Autodesk Fusion 360 part; units mm, degrees
(part 3 of 4)
sketch "Sketch19" plane through (0, 0, 6.5) normal (0, 0, 1) x (-1, 0, 0)
  line L0 (61.5, -17) -> (61.5, 17)
  arc A0 (63.5, 19) -> (61.5, 17) centre (63.5, 17) ccw
  line L1 (63.5, 19) -> (68.5, 19)
  arc A1 (70.5, 17) -> (68.5, 19) centre (68.5, 17) ccw
  line L2 (70.5, 17) -> (70.5, -17)
  arc A2 (68.5, -19) -> (70.5, -17) centre (68.5, -17) ccw
  line L3 (68.5, -19) -> (63.5, -19)
  arc A3 (61.5, -17) -> (63.5, -19) centre (63.5, -17) ccw
  line L4 (59.5, 16.3) -> (20.05, 16.3)
  line L5 (20.05, 16.3) -> (20.05, 38.6)
  arc A4 (20.05, 38.6) -> (18.05, 40.6) centre (18.05, 38.6) ccw
  line L6 (18.05, 40.6) -> (-18.05, 40.6)
  arc A5 (-18.05, 40.6) -> (-20.05, 38.6) centre (-18.05, 38.6) ccw
  line L7 (-20.05, 38.6) -> (-20.05, 16.3)
  line L8 (-20.05, 16.3) -> (-72.5, 16.3)
  line L9 (-72.5, 16.3) -> (-72.5, -16.3)
  line L10 (-72.5, -16.3) -> (-20.05, -16.3)
  line L11 (-20.05, -16.3) -> (-20.05, -38.6)
  arc A6 (-20.05, -38.6) -> (-18.05, -40.6) centre (-18.05, -38.6) ccw
  line L12 (-18.05, -40.6) -> (18.05, -40.6)
  arc A7 (18.05, -40.6) -> (20.05, -38.6) centre (18.05, -38.6) ccw
  line L13 (20.05, -38.6) -> (20.05, -16.3)
  line L14 (20.05, -16.3) -> (59.5, -16.3)
  line L15 (59.5, -16.3) -> (59.5, -28.9174)
  arc A8 (61.5, -28.5) -> (59.5, -28.9174) centre (61.5, -33.5) ccw
  line L16 (61.5, -28.5) -> (72.5, -28.5)
  line L17 (72.5, -28.5) -> (72.5, 28.5)
  line L18 (72.5, 28.5) -> (61.5, 28.5)
  arc A9 (59.5, 28.9174) -> (61.5, 28.5) centre (61.5, 33.5) ccw
  line L19 (59.5, 28.9174) -> (59.5, 16.3)
  circle A10 centre (-10, 34.75) radius 2.425
  circle A11 centre (10, -34.75) radius 2.425
  circle A12 centre (-10, -34.75) radius 2.425
  circle A13 centre (10, 34.75) radius 2.425
  line L20 (59.5, -8.8707) -> (59.5, 8.8707)
  line L21 (-70.5, -8.9444) -> (-70.5, 8.9444)
  line L22 (55.628, -14.3) -> (-65.7592, -14.3)
  line L23 (55.628, 14.3) -> (-65.7592, 14.3)
  line L24 (55.7295, 13.3104) -> (1.8744, 2.1388)
  line L25 (-1.8855, 2.081) -> (-65.8457, 13.3075)
  line L26 (-68.1756, 10.918) -> (-4.7518, 0.4934)
  line L27 (-4.7518, -0.4934) -> (-68.1756, -10.918)
  line L28 (-65.8457, -13.3075) -> (-1.8855, -2.081)
  line L29 (1.8744, -2.1388) -> (55.7295, -13.3104)
  line L30 (57.1159, -10.8335) -> (4.2578, -0.4907)
  line L31 (4.2578, 0.4907) -> (57.1159, 10.8335)
  arc A14 (55.628, -14.3) -> (55.7295, -13.3104) centre (55.628, -13.8) ccw
  arc A15 (-65.8457, -13.3075) -> (-65.7592, -14.3) centre (-65.7592, -13.8) ccw
  arc A16 (-65.7592, 14.3) -> (-65.8457, 13.3075) centre (-65.7592, 13.8) ccw
  arc A17 (55.7295, 13.3104) -> (55.628, 14.3) centre (55.628, 13.8) ccw
  arc A18 (57.1159, -10.8335) -> (59.5, -8.8707) centre (57.5, -8.8707) ccw
  arc A19 (59.5, 8.8707) -> (57.1159, 10.8335) centre (57.5, 8.8707) ccw
  arc A20 (-68.1756, 10.918) -> (-70.5, 8.9444) centre (-68.5, 8.9444) ccw
  arc A21 (-70.5, -8.9444) -> (-68.1756, -10.918) centre (-68.5, -8.9444) ccw
  arc A22 (-1.8855, 2.081) -> (1.8744, 2.1388) centre (-0.1567, 11.9304) ccw
  arc A23 (1.8744, -2.1388) -> (-1.8855, -2.081) centre (-0.1567, -11.9304) ccw
  arc A24 (-4.7518, -0.4934) -> (-4.7518, 0.4934) centre (-4.8329, 0) ccw
  arc A25 (4.2578, 0.4907) -> (4.2578, -0.4907) centre (4.3538, 0) ccw
  point P0 (-70.5, -11.3)
  point P1 (-70.5, 11.3)
  point P2 (60.5, 14.3)
  point P3 (-71.5, 14.3)
  point P4 (0, 1.75)
  point P5 (-1.75, 0)
  point P6 (0, -1.75)
  point P7 (1.75, 0)
  dimension "d143" = 2
  dimension "d144" = 2
  dimension "d145" = 5
  dimension "d146" = 5
  dimension "d147" = 2
  dimension "d148" = 2
  dimension "d149" = 1
  dimension "d150" = 1
  dimension "d151" = 3.5
  dimension "d152" = 3.5
  dimension "d153" = 1.75
  dimension "d154" = 1.75
  dimension "d155" = 0.5
  dimension "d156" = 2
  dimension "d157" = 10
  dimension "d158" = 0.5
  constraint perpendicular L14 L20
  constraint perpendicular L8 L21
  constraint perpendicular L15 L22
  constraint perpendicular L21 L23
  constraint vertical P4 P6
  constraint vertical origin P4
  constraint horizontal P5 P7
  constraint horizontal origin P7
  constraint tangent L22 A14
  constraint tangent L29 A14
  constraint tangent L28 A15
  constraint tangent L22 A15
  constraint equal A14 A15
  constraint coincident P3 L25
  constraint coincident P3 L23
  constraint tangent L25 A16
  constraint tangent L23 A16
  constraint equal A14 A16
  constraint coincident P2 L23
  constraint coincident P2 L24
  constraint tangent L23 A17
  constraint tangent L24 A17
  constraint equal A14 A17
  constraint tangent L30 A18
  constraint tangent L20 A18
  constraint tangent L20 A19
  constraint tangent L31 A19
  constraint equal A18 A19
  constraint coincident P1 L26
  constraint coincident P1 L21
  constraint tangent L26 A20
  constraint tangent L21 A20
  constraint equal A18 A20
  constraint coincident P0 L21
  constraint coincident P0 L27
  constraint tangent L21 A21
  constraint tangent L27 A21
  constraint equal A18 A21
  constraint tangent L24 A22
  constraint tangent L25 A22
  constraint tangent L29 A23
  constraint tangent L28 A23
  constraint equal A22 A23
  constraint tangent L27 A24
  constraint tangent L26 A24
  constraint tangent L31 A25
  constraint tangent L30 A25
  constraint equal A24 A25
  measures "d143" distance of L0 L20
  measures "d144" distance of L9 L21
  measures "d145" distance of L10 P0
  measures "d146" distance of L8 P1
  measures "d147" distance of L4 L23
  measures "d148" distance of L14 L22
  measures "d149" distance of L9 P3
  measures "d150" distance of L0 P2
  measures "d151" distance of P4 P6
  measures "d152" distance of P5 P7
  measures "d153" distance of origin P4
  measures "d154" distance of origin P5
  measures "d155" radius of A14
  measures "d157" radius of A22
  measures "d158" radius of A24
extrude "Extrude21" cut sketch "Sketch19" against normal blind 6.5 contours L20 L30 L31 A18 A19 A25 | L21 L26 L27 A20 A21 A24 | L22 L28 L29 A14 A15 A23 | L23 L24 L25 A16 A17 A22
sketch "Sketch20" plane through (0, 0, 6.5) normal (0, 0, 1) x (-1, 0, 0)
  line L0 (-4.7518, -0.4934) -> (-68.1756, -10.918)
  arc A0 (-70.5, -8.9444) -> (-68.1756, -10.918) centre (-68.5, -8.9444) ccw
  line L1 (-70.5, -8.9444) -> (-70.5, 8.9444)
  arc A1 (-68.1756, 10.918) -> (-70.5, 8.9444) centre (-68.5, 8.9444) ccw
  line L2 (-68.1756, 10.918) -> (-4.7518, 0.4934)
  arc A2 (-4.7518, -0.4934) -> (-4.7518, 0.4934) centre (-4.8329, 0) ccw
  line L3 (59.5, 8.8707) -> (59.5, -8.8707)
  arc A3 (57.1159, -10.8335) -> (59.5, -8.8707) centre (57.5, -8.8707) ccw
  line L4 (57.1159, -10.8335) -> (4.2578, -0.4907)
  arc A4 (4.2578, 0.4907) -> (4.2578, -0.4907) centre (4.3538, 0) ccw
  line L5 (4.2578, 0.4907) -> (57.1159, 10.8335)
  arc A5 (59.5, 8.8707) -> (57.1159, 10.8335) centre (57.5, 8.8707) ccw
  line L6 (-65.7592, 14.3) -> (55.628, 14.3)
  arc A6 (55.7295, 13.3104) -> (55.628, 14.3) centre (55.628, 13.8) ccw
  line L7 (55.7295, 13.3104) -> (1.8744, 2.1388)
  arc A7 (-1.8855, 2.081) -> (1.8744, 2.1388) centre (-0.1567, 11.9304) ccw
  line L8 (-1.8855, 2.081) -> (-65.8457, 13.3075)
  arc A8 (-65.7592, 14.3) -> (-65.8457, 13.3075) centre (-65.7592, 13.8) ccw
  line L9 (1.8744, -2.1388) -> (55.7295, -13.3104)
  arc A9 (55.628, -14.3) -> (55.7295, -13.3104) centre (55.628, -13.8) ccw
  line L10 (55.628, -14.3) -> (-65.7592, -14.3)
  arc A10 (-65.8457, -13.3075) -> (-65.7592, -14.3) centre (-65.7592, -13.8) ccw
  line L11 (-65.8457, -13.3075) -> (-1.8855, -2.081)
  arc A11 (1.8744, -2.1388) -> (-1.8855, -2.081) centre (-0.1567, -11.9304) ccw
  line L12 (61.5, -17) -> (61.5, 17)
  arc A12 (63.5, 19) -> (61.5, 17) centre (63.5, 17) ccw
  line L13 (63.5, 19) -> (68.5, 19)
  arc A13 (70.5, 17) -> (68.5, 19) centre (68.5, 17) ccw
  line L14 (70.5, 17) -> (70.5, -17)
  arc A14 (68.5, -19) -> (70.5, -17) centre (68.5, -17) ccw
  line L15 (68.5, -19) -> (63.5, -19)
  arc A15 (61.5, -17) -> (63.5, -19) centre (63.5, -17) ccw
  line L16 (59.5, 16.3) -> (20.05, 16.3)
  line L17 (20.05, 16.3) -> (20.05, 38.6)
  arc A16 (20.05, 38.6) -> (18.05, 40.6) centre (18.05, 38.6) ccw
  line L18 (18.05, 40.6) -> (-18.05, 40.6)
  arc A17 (-18.05, 40.6) -> (-20.05, 38.6) centre (-18.05, 38.6) ccw
  line L19 (-20.05, 38.6) -> (-20.05, 16.3)
  line L20 (-20.05, 16.3) -> (-72.5, 16.3)
  line L21 (-72.5, 16.3) -> (-72.5, -16.3)
  line L22 (-72.5, -16.3) -> (-20.05, -16.3)
  line L23 (-20.05, -16.3) -> (-20.05, -38.6)
  arc A18 (-20.05, -38.6) -> (-18.05, -40.6) centre (-18.05, -38.6) ccw
  line L24 (-18.05, -40.6) -> (18.05, -40.6)
  arc A19 (18.05, -40.6) -> (20.05, -38.6) centre (18.05, -38.6) ccw
  line L25 (20.05, -38.6) -> (20.05, -16.3)
  line L26 (20.05, -16.3) -> (59.5, -16.3)
  line L27 (59.5, -16.3) -> (59.5, -28.9174)
  arc A20 (61.5, -28.5) -> (59.5, -28.9174) centre (61.5, -33.5) ccw
  line L28 (61.5, -28.5) -> (72.5, -28.5)
  line L29 (72.5, -28.5) -> (72.5, 28.5)
  line L30 (72.5, 28.5) -> (61.5, 28.5)
  arc A21 (59.5, 28.9174) -> (61.5, 28.5) centre (61.5, 33.5) ccw
  line L31 (59.5, 28.9174) -> (59.5, 16.3)
  circle A22 centre (-10, 34.75) radius 2.425
  circle A23 centre (10, -34.75) radius 2.425
  circle A24 centre (-10, -34.75) radius 2.425
  circle A25 centre (10, 34.75) radius 2.425
  line L32 (16.05, 16.3) -> (-16.05, 16.3)
  line L33 (-18.05, 18.3) -> (-18.05, 28.325)
  line L34 (-16.05, 30.325) -> (-7.575, 30.325)
  line L35 (18.05, 28.325) -> (18.05, 18.3)
  line L36 (-7.575, -30.325) -> (-16.05, -30.325)
  line L37 (-18.05, -28.325) -> (-18.05, -18.3)
  line L38 (-16.05, -16.3) -> (16.05, -16.3)
  line L39 (18.05, -18.3) -> (18.05, -28.325)
  arc A26 (16.05, 16.3) -> (18.05, 18.3) centre (16.05, 18.3) ccw
  arc A27 (18.05, 28.325) -> (16.05, 30.325) centre (16.05, 28.325) ccw
  arc A28 (-16.05, 30.325) -> (-18.05, 28.325) centre (-16.05, 28.325) ccw
  arc A29 (-18.05, 18.3) -> (-16.05, 16.3) centre (-16.05, 18.3) ccw
  arc A30 (18.05, -18.3) -> (16.05, -16.3) centre (16.05, -18.3) ccw
  arc A31 (16.05, -30.325) -> (18.05, -28.325) centre (16.05, -28.325) ccw
  arc A32 (-18.05, -28.325) -> (-16.05, -30.325) centre (-16.05, -28.325) ccw
  arc A33 (-16.05, -16.3) -> (-18.05, -18.3) centre (-16.05, -18.3) ccw
  line L40 (5.575, -32.325) -> (5.575, -38.6)
  line L41 (3.575, -40.6) -> (-3.575, -40.6)
  line L42 (-5.575, -38.6) -> (-5.575, -32.325)
  arc A34 (-5.575, -32.325) -> (-7.575, -30.325) centre (-7.575, -32.325) ccw
  line L43 (16.05, -30.325) -> (7.575, -30.325)
  arc A35 (7.575, -30.325) -> (5.575, -32.325) centre (7.575, -32.325) ccw
  arc A36 (-5.575, -38.6) -> (-3.575, -40.6) centre (-3.575, -38.6) ccw
  arc A37 (3.575, -40.6) -> (5.575, -38.6) centre (3.575, -38.6) ccw
  line L44 (-5.575, 30.325) -> (5.575, 30.325)
  line L45 (5.575, 32.325) -> (5.575, 38.6)
  line L46 (3.575, 40.6) -> (-3.575, 40.6)
  line L47 (-5.575, 38.6) -> (-5.575, 32.325)
  arc A38 (-3.575, 40.6) -> (-5.575, 38.6) centre (-3.575, 38.6) ccw
  arc A39 (5.575, 38.6) -> (3.575, 40.6) centre (3.575, 38.6) ccw
  arc A40 (-7.575, 30.325) -> (-5.575, 32.325) centre (-7.575, 32.325) ccw
  line L48 (7.575, 30.325) -> (16.05, 30.325)
  arc A41 (5.575, 32.325) -> (7.575, 30.325) centre (7.575, 32.325) ccw
  line L49 (-67.5, 42.6) -> (51.5, 42.6)
  line L50 (51.5, -42.6) -> (-67.5, -42.6)
  dimension "d161" = 4.425
  dimension "d162" = 4.425
  dimension "d163" = 2
  dimension "d164" = 2
  dimension "d165" = 2
  dimension "d166" = 2
  dimension "d167" = 2
  dimension "d168" = 2
  dimension "d215" = 4.425
  dimension "d216" = 4.425
  dimension "d218" = 2
  dimension "d219" = 2
  dimension "d220" = 2
  dimension "d221" = 4.425
  dimension "d222" = 4.425
  dimension "d224" = 2
  dimension "d225" = 2
  dimension "d226" = 2
  dimension "d254" = 2
  dimension "d255" = 2
  constraint horizontal L32
  constraint vertical L33
  constraint horizontal L34
  constraint vertical L35
  constraint horizontal L36
  constraint vertical L37
  constraint horizontal L38
  constraint vertical L39
  constraint tangent L32 A26
  constraint tangent L35 A26
  constraint tangent L35 A27
  constraint tangent L34 A27
  constraint equal A26 A27
  constraint tangent L34 A28
  constraint tangent L33 A28
  constraint equal A26 A28
  constraint tangent L33 A29
  constraint tangent L32 A29
  constraint equal A26 A29
  constraint tangent L38 A30
  constraint tangent L39 A30
  constraint tangent L39 A31
  constraint tangent L36 A31
  constraint equal A30 A31
  constraint tangent L36 A32
  constraint tangent L37 A32
  constraint equal A30 A32
  constraint tangent L37 A33
  constraint tangent L38 A33
  constraint equal A30 A33
  constraint vertical L40
  constraint horizontal L41
  constraint vertical L42
  constraint coincident L36 A31.start
  constraint tangent L42 A34
  constraint tangent L36 A34
  constraint tangent A31 L43
  constraint tangent L40 A35
  constraint tangent L43 A35
  constraint tangent L42 A36
  constraint tangent L41 A36
  constraint tangent L41 A37
  constraint tangent L40 A37
  constraint equal A36 A37
  constraint horizontal L44
  constraint vertical L45
  constraint horizontal L46
  constraint vertical L47
  constraint coincident L34 L44.start
  constraint tangent L47 A38
  constraint tangent L46 A38
  constraint tangent L46 A39
  constraint tangent L45 A39
  constraint equal A38 A39
  constraint coincident L44.start L47
  constraint tangent L47 A40
  constraint tangent L34 A40
  constraint tangent A27 L48
  constraint coincident L44.end L45
  constraint coincident L44.end L48
  constraint tangent L45 A41
  constraint tangent L48 A41
  measures "d161" distance of A25.centre L34
  measures "d162" distance of A23.centre L36
  measures "d163" distance of L25 L39
  measures "d164" distance of L23 L37
  measures "d165" distance of L6 L32
  measures "d166" distance of L10 L38
  measures "d167" radius of A26
  measures "d168" radius of A30
  measures "d215" distance of A23.centre L40
  measures "d216" distance of A24.centre L42
  measures "d218" radius of A34
  measures "d219" radius of A35
  measures "d220" radius of A36
  measures "d221" distance of A25.centre L45
  measures "d222" distance of A22.centre L47
  measures "d224" radius of A38
  measures "d225" radius of A40
  measures "d226" radius of A41
  measures "d254" distance of L46 L49
  measures "d255" distance of L41 L50
extrude "Extrude22" cut sketch "Sketch20" against normal blind 6.5 contours L18 L32 L33 L34 L35 A26 A27 A28 A29 L45 L46 L47 A38 A39 A40 L48 A41 | L24 L36 L37 L38 L39 A30 A31 A32 A33 L40 L41 L42 A34 L43 A35 A36 A37
ref_plane "WorkPlane3" through (8, -36.725, 15) normal (0, 0, 1) x (1, 0, 0)
sketch "Sketch21" plane through (0, 0, 15) normal (0, 0, 1) x (1, 0, 0)
  line L0 (-41.4565, -30.974) -> (-24.05, -30.974)
  line L1 (-22.05, -32.974) -> (-22.05, -38.6)
  line L2 (-24.05, -40.6) -> (-41.4565, -40.6)
  line L3 (-43.4565, -38.6) -> (-43.4565, -32.974)
  line L4 (24.05, -30.974) -> (57.4565, -30.974)
  line L5 (59.4565, -32.974) -> (59.4565, -38.6)
  line L6 (57.4565, -40.6) -> (24.05, -40.6)
  line L7 (22.05, -38.6) -> (22.05, -32.974)
  line L8 (-41.4565, 40.6) -> (-24.05, 40.6)
  line L9 (-22.05, 38.6) -> (-22.05, 32.974)
  line L10 (-24.05, 30.974) -> (-41.4565, 30.974)
  line L11 (-43.4565, 32.974) -> (-43.4565, 38.6)
  line L12 (24.05, 40.6) -> (57.4565, 40.6)
  line L13 (59.4565, 38.6) -> (59.4565, 32.974)
  line L14 (57.4565, 30.974) -> (24.05, 30.974)
  line L15 (22.05, 32.974) -> (22.05, 38.6)
  line L16 (67.5, -42.6) -> (-51.5, -42.6)
  line L17 (-51.5, 42.6) -> (67.5, 42.6)
  line L18 (-20.05, -33.5) -> (-20.05, -38.6)
  line L19 (20.05, 33.5) -> (20.05, 38.6)
  line L20 (-56.5, -28.974) -> (-20.05, -28.974)
  line L21 (-20.05, 28.974) -> (-56.5, 28.974)
  circle A0 centre (-49, -35.1) radius 3.5435
  circle A1 centre (65, 35.1) radius 3.5435
  arc A2 (-41.4565, 40.6) -> (-43.4565, 38.6) centre (-41.4565, 38.6) ccw
  arc A3 (-22.05, 38.6) -> (-24.05, 40.6) centre (-24.05, 38.6) ccw
  arc A4 (-24.05, 30.974) -> (-22.05, 32.974) centre (-24.05, 32.974) ccw
  arc A5 (-43.4565, 32.974) -> (-41.4565, 30.974) centre (-41.4565, 32.974) ccw
  arc A6 (24.05, 40.6) -> (22.05, 38.6) centre (24.05, 38.6) ccw
  arc A7 (59.4565, 38.6) -> (57.4565, 40.6) centre (57.4565, 38.6) ccw
  arc A8 (57.4565, 30.974) -> (59.4565, 32.974) centre (57.4565, 32.974) ccw
  arc A9 (22.05, 32.974) -> (24.05, 30.974) centre (24.05, 32.974) ccw
  arc A10 (-41.4565, -30.974) -> (-43.4565, -32.974) centre (-41.4565, -32.974) ccw
  arc A11 (-22.05, -32.974) -> (-24.05, -30.974) centre (-24.05, -32.974) ccw
  arc A12 (-24.05, -40.6) -> (-22.05, -38.6) centre (-24.05, -38.6) ccw
  arc A13 (-43.4565, -38.6) -> (-41.4565, -40.6) centre (-41.4565, -38.6) ccw
  arc A14 (24.05, -30.974) -> (22.05, -32.974) centre (24.05, -32.974) ccw
  arc A15 (59.4565, -32.974) -> (57.4565, -30.974) centre (57.4565, -32.974) ccw
  arc A16 (57.4565, -40.6) -> (59.4565, -38.6) centre (57.4565, -38.6) ccw
  arc A17 (22.05, -38.6) -> (24.05, -40.6) centre (24.05, -38.6) ccw
  dimension "d172" = 2
  dimension "d173" = 2
  dimension "d174" = 2
  dimension "d175" = 2
  dimension "d176" = 2
  dimension "d177" = 2
  dimension "d178" = 5.5435
  dimension "d179" = 5.5435
  dimension "d180" = 2
  dimension "d181" = 2
  dimension "d182" = 2
  dimension "d183" = 2
  constraint horizontal L0
  constraint vertical L1
  constraint horizontal L2
  constraint vertical L3
  constraint horizontal L4
  constraint vertical L5
  constraint horizontal L6
  constraint vertical L7
  constraint horizontal L8
  constraint vertical L9
  constraint horizontal L10
  constraint vertical L11
  constraint horizontal L12
  constraint vertical L13
  constraint horizontal L14
  constraint vertical L15
  constraint tangent L8 A2
  constraint tangent L11 A2
  constraint tangent L8 A3
  constraint tangent L9 A3
  constraint equal A2 A3
  constraint tangent L9 A4
  constraint tangent L10 A4
  constraint equal A2 A4
  constraint tangent L10 A5
  constraint tangent L11 A5
  constraint equal A2 A5
  constraint tangent L15 A6
  constraint tangent L12 A6
  constraint tangent L12 A7
  constraint tangent L13 A7
  constraint equal A6 A7
  constraint tangent L13 A8
  constraint tangent L14 A8
  constraint equal A6 A8
  constraint tangent L14 A9
  constraint tangent L15 A9
  constraint equal A6 A9
  constraint tangent L3 A10
  constraint tangent L0 A10
  constraint tangent L0 A11
  constraint tangent L1 A11
  constraint equal A10 A11
  constraint tangent L1 A12
  constraint tangent L2 A12
  constraint equal A10 A12
  constraint tangent L2 A13
  constraint tangent L3 A13
  constraint equal A10 A13
  constraint tangent L7 A14
  constraint tangent L4 A14
  constraint tangent L4 A15
  constraint tangent L5 A15
  constraint equal A14 A15
  constraint tangent L5 A16
  constraint tangent L6 A16
  constraint equal A14 A16
  constraint tangent L6 A17
  constraint tangent L7 A17
  constraint equal A14 A17
  constraint vertical A8.centre A15.centre
  constraint vertical A9.centre A14.centre
  constraint horizontal A11.centre A14.centre
  constraint horizontal A12.centre A17.centre
  constraint vertical A4.centre A11.centre
  constraint vertical A5.centre A10.centre
  constraint horizontal A4.centre A9.centre
  constraint horizontal A3.centre A6.centre
  measures "d172" distance of L2 L16
  measures "d173" distance of L8 L17
  measures "d174" distance of L1 L18
  measures "d175" distance of L15 L19
  measures "d176" distance of L0 L20
  measures "d177" distance of L10 L21
  measures "d178" distance of L3 A0.centre
  measures "d179" distance of L13 A1.centre
  measures "d180" radius of A2
  measures "d181" radius of A6
  measures "d182" radius of A10
  measures "d183" radius of A14
extrude "Extrude23" cut sketch "Sketch21" against normal blind 15 contours L0 L1 L2 L3 A10 A11 A12 A13 | L4 L5 L6 L7 A14 A15 A16 A17 | L8 L9 L10 L11 A2 A3 A4 A5 | L12 L13 L14 L15 A6 A7 A8 A9
sketch "Sketch22" plane through (-72.5, 0, 0) normal (-1, 0, 0) x (0, -1, 0)
  line L0 (-28.5, 6.5) -> (-28.5, 0)
  line L1 (-28.5, 0) -> (28.5, 0)
  line L2 (28.5, 0) -> (28.5, 6.5)
  line L3 (28.5, 6.5) -> (-28.5, 6.5)
  line L4 (-18, 4.5) -> (18, 4.5)
  line L5 (19, 3.5) -> (19, 3)
  line L6 (18, 2) -> (-18, 2)
  line L7 (-19, 3) -> (-19, 3.5)
  arc A0 (-18, 4.5) -> (-19, 3.5) centre (-18, 3.5) ccw
  arc A1 (-19, 3) -> (-18, 2) centre (-18, 3) ccw
  arc A2 (18, 2) -> (19, 3) centre (18, 3) ccw
  arc A3 (19, 3.5) -> (18, 4.5) centre (18, 3.5) ccw
  dimension "d186" = 2
  dimension "d187" = 2
  dimension "d190" = 1
  dimension "d287" = 9.5
  dimension "d288" = 9.5
  constraint horizontal L4
  constraint vertical L5
  constraint horizontal L6
  constraint vertical L7
  constraint tangent L4 A0
  constraint tangent L7 A0
  constraint tangent L7 A1
  constraint tangent L6 A1
  constraint equal A0 A1
  constraint tangent L6 A2
  constraint tangent L5 A2
  constraint equal A0 A2
  constraint tangent L5 A3
  constraint tangent L4 A3
  constraint equal A0 A3
  measures "d186" distance of L3 L4
  measures "d187" distance of L1 L6
  measures "d190" radius of A0
  measures "d287" distance of L2 L5
  measures "d288" distance of L0 L7
extrude "Extrude24" cut sketch "Sketch22" against normal blind 5 contours L4 L5 L6 L7 A0 A1 A2 A3
sketch "Sketch23" plane through (-61.5, 0, 0) normal (-1, 0, 0) x (0, -1, 0)
  line L0 (17, 6.5) -> (-17, 6.5)
  line L1 (-17, 6.5) -> (-17, 0)
  line L2 (-17, 0) -> (17, 0)
  line L3 (17, 0) -> (17, 6.5)
  line L4 (-9, 4.5) -> (9, 4.5)
  line L5 (10, 3.5) -> (10, 3)
  line L6 (9, 2) -> (-9, 2)
  line L7 (-10, 3) -> (-10, 3.5)
  arc A0 (-9, 4.5) -> (-10, 3.5) centre (-9, 3.5) ccw
  arc A1 (-10, 3) -> (-9, 2) centre (-9, 3) ccw
  arc A2 (9, 2) -> (10, 3) centre (9, 3) ccw
  arc A3 (10, 3.5) -> (9, 4.5) centre (9, 3.5) ccw
  dimension "d193" = 20
  dimension "d194" = 10
  dimension "d195" = 2
  dimension "d196" = 2
  dimension "d197" = 1
  constraint horizontal L4
  constraint vertical L5
  constraint horizontal L6
  constraint vertical L7
  constraint tangent L4 A0
  constraint tangent L7 A0
  constraint tangent L7 A1
  constraint tangent L6 A1
  constraint equal A0 A1
  constraint tangent L6 A2
  constraint tangent L5 A2
  constraint equal A0 A2
  constraint tangent L5 A3
  constraint tangent L4 A3
  constraint equal A0 A3
  measures "d193" distance of L5 L7
  measures "d194" distance of origin L7
  measures "d195" distance of L2 L6
  measures "d196" distance of L0 L4
  measures "d197" radius of A0
extrude "Extrude25" cut sketch "Sketch23" against normal blind 5 contours L4 L5 L6 L7 A0 A1 A2 A3
sketch "Sketch24" plane through (72.5, 0, 0) normal (1, 0, 0) x (0, 1, 0)
  line L0 (37.6, 0) -> (37.6, 10)
  line L1 (37.6, 10) -> (33.5, 10)
  arc A0 (28.974, 12.875) -> (33.5, 10) centre (33.5, 15) ccw
  arc A1 (28.974, 12.875) -> (24.4481, 15.75) centre (24.4481, 10.75) ccw
  line L2 (24.4481, 15.75) -> (24.3, 15.75)
  arc A2 (24.3, 15.75) -> (19.3, 10.75) centre (24.3, 10.75) ccw
  line L3 (19.3, 10.75) -> (19.3, 9.5)
  arc A3 (16.3, 6.5) -> (19.3, 9.5) centre (16.3, 9.5) ccw
  line L4 (16.3, 6.5) -> (-16.3, 6.5)
  arc A4 (-19.3, 9.5) -> (-16.3, 6.5) centre (-16.3, 9.5) ccw
  line L5 (-19.3, 9.5) -> (-19.3, 10.75)
  arc A5 (-19.3, 10.75) -> (-24.3, 15.75) centre (-24.3, 10.75) ccw
  line L6 (-24.3, 15.75) -> (-24.4481, 15.75)
  arc A6 (-24.4481, 15.75) -> (-28.974, 12.875) centre (-24.4481, 10.75) ccw
  arc A7 (-33.5, 10) -> (-28.974, 12.875) centre (-33.5, 15) ccw
  line L7 (-33.5, 10) -> (-37.6, 10)
  line L8 (-37.6, 10) -> (-37.6, 0)
  line L9 (-37.6, 0) -> (37.6, 0)
  line L10 (-9, 4.5) -> (9, 4.5)
  line L11 (10, 3.5) -> (10, 3)
  line L12 (9, 2) -> (-9, 2)
  line L13 (-10, 3) -> (-10, 3.5)
  arc A8 (-9, 4.5) -> (-10, 3.5) centre (-9, 3.5) ccw
  arc A9 (-10, 3) -> (-9, 2) centre (-9, 3) ccw
  arc A10 (9, 2) -> (10, 3) centre (9, 3) ccw
  arc A11 (10, 3.5) -> (9, 4.5) centre (9, 3.5) ccw
  dimension "d200" = 2
  dimension "d201" = 2
  dimension "d202" = 10
  dimension "d203" = 20
  dimension "d204" = 1
  constraint horizontal L10
  constraint vertical L11
  constraint horizontal L12
  constraint vertical L13
  constraint tangent L10 A8
  constraint tangent L13 A8
  constraint tangent L13 A9
  constraint tangent L12 A9
  constraint equal A8 A9
  constraint tangent L12 A10
  constraint tangent L11 A10
  constraint equal A8 A10
  constraint tangent L11 A11
  constraint tangent L10 A11
  constraint equal A8 A11
  measures "d200" distance of L4 L10
  measures "d201" distance of L9 L12
  measures "d202" distance of origin L11
  measures "d203" distance of L11 L13
  measures "d204" radius of A8
extrude "Extrude26" cut sketch "Sketch24" against normal blind 5 contours L10 L11 L12 L13 A8 A9 A10 A11
sketch "Sketch25" plane through (0, 14.3, 0) normal (0, -1, 0) x (1, 0, 0)
  line L0 (65.7592, 6.5) -> (-55.628, 6.5)
  line L1 (-55.628, 6.5) -> (-55.628, 0)
  line L2 (-55.628, 0) -> (65.7592, 0)
  line L3 (65.7592, 0) -> (65.7592, 6.5)
  line L4 (-17.05, 4.5) -> (17.05, 4.5)
  line L5 (18.05, 3.5) -> (18.05, 3)
  line L6 (17.05, 2) -> (-17.05, 2)
  line L7 (-18.05, 3) -> (-18.05, 3.5)
  line L8 (67.5, 10) -> (-51.5, 10)
  arc A0 (-17.05, 4.5) -> (-18.05, 3.5) centre (-17.05, 3.5) ccw
  arc A1 (-18.05, 3) -> (-17.05, 2) centre (-17.05, 3) ccw
  arc A2 (17.05, 2) -> (18.05, 3) centre (17.05, 3) ccw
  arc A3 (18.05, 3.5) -> (17.05, 4.5) centre (17.05, 3.5) ccw
  dimension "d207" = 36.1
  dimension "d208" = 18.05
  dimension "d209" = 2
  dimension "d211" = 1
  dimension "d212" = 2
  constraint horizontal L4
  constraint vertical L5
  constraint horizontal L6
  constraint vertical L7
  constraint tangent L4 A0
  constraint tangent L7 A0
  constraint tangent L7 A1
  constraint tangent L6 A1
  constraint equal A0 A1
  constraint tangent L6 A2
  constraint tangent L5 A2
  constraint equal A0 A2
  constraint tangent L5 A3
  constraint tangent L4 A3
  constraint equal A0 A3
  measures "d207" distance of L5 L7
  measures "d208" distance of origin L5
  measures "d209" distance of L2 L6
  measures "d211" radius of A0
  measures "d212" distance of L0 L4
extrude "Extrude27" cut sketch "Sketch25" against normal blind 5 contours L4 L5 L6 L7 A0 A1 A2 A3
sketch "Sketch26" plane through (0, -14.3, 0) normal (0, 1, 0) x (-1, 0, 0)
  line L0 (55.628, 6.5) -> (-65.7592, 6.5)
  line L1 (-65.7592, 6.5) -> (-65.7592, 0)
  line L2 (-65.7592, 0) -> (55.628, 0)
  line L3 (55.628, 0) -> (55.628, 6.5)
  line L4 (-17.05, 4.5) -> (17.05, 4.5)
  line L5 (18.05, 3.5) -> (18.05, 3)
  line L6 (17.05, 2) -> (-17.05, 2)
  line L7 (-18.05, 3) -> (-18.05, 3.5)
  arc A0 (-17.05, 4.5) -> (-18.05, 3.5) centre (-17.05, 3.5) ccw
  arc A1 (18.05, 3.5) -> (17.05, 4.5) centre (17.05, 3.5) ccw
  arc A2 (17.05, 2) -> (18.05, 3) centre (17.05, 3) ccw
  arc A3 (-18.05, 3) -> (-17.05, 2) centre (-17.05, 3) ccw
  dimension "d227" = 2
  dimension "d228" = 2
  dimension "d229" = 36.1
  dimension "d230" = 18.05
  dimension "d231" = 1
  constraint horizontal L4
  constraint vertical L5
  constraint horizontal L6
  constraint vertical L7
  constraint tangent L7 A0
  constraint tangent L4 A0
  constraint tangent L4 A1
  constraint tangent L5 A1
  constraint equal A0 A1
  constraint tangent L5 A2
  constraint tangent L6 A2
  constraint equal A0 A2
  constraint tangent L6 A3
  constraint tangent L7 A3
  constraint equal A0 A3
  measures "d227" distance of L0 L4
  measures "d228" distance of L2 L6
  measures "d229" distance of L5 L7
  measures "d230" distance of origin L5
  measures "d231" radius of A0
extrude "Extrude28" cut sketch "Sketch26" against normal blind 5 contours L4 L5 L6 L7 A0 A1 A2 A3
sketch "Sketch27" plane through (0, -42.6, 0) normal (0, -1, 0) x (1, 0, 0)
  line L0 (67.5, 0) -> (67.5, 10)
  line L1 (67.5, 10) -> (-51.5, 10)
  line L2 (-51.5, 10) -> (-51.5, 0)
  line L3 (-51.5, 0) -> (67.5, 0)
  line L4 (-41.4565, 8) -> (-24.05, 8)
  line L5 (-22.05, 6) -> (-22.05, 4)
  line L6 (-24.05, 2) -> (-41.4565, 2)
  line L7 (-43.4565, 4) -> (-43.4565, 6)
  line L8 (24.05, 8) -> (57.4565, 8)
  line L9 (59.4565, 6) -> (59.4565, 4)
  line L10 (57.4565, 2) -> (24.05, 2)
  line L11 (22.05, 4) -> (22.05, 6)
  arc A0 (-41.4565, 8) -> (-43.4565, 6) centre (-41.4565, 6) ccw
  arc A1 (-43.4565, 4) -> (-41.4565, 2) centre (-41.4565, 4) ccw
  arc A2 (-24.05, 2) -> (-22.05, 4) centre (-24.05, 4) ccw
  arc A3 (-22.05, 6) -> (-24.05, 8) centre (-24.05, 6) ccw
  arc A4 (24.05, 8) -> (22.05, 6) centre (24.05, 6) ccw
  arc A5 (59.4565, 6) -> (57.4565, 8) centre (57.4565, 6) ccw
  arc A6 (57.4565, 2) -> (59.4565, 4) centre (57.4565, 4) ccw
  arc A7 (22.05, 4) -> (24.05, 2) centre (24.05, 4) ccw
  line L12 (-3.575, 8) -> (3.575, 8)
  line L13 (5.575, 6) -> (5.575, 4)
  line L14 (3.575, 2) -> (-3.575, 2)
  line L15 (-5.575, 4) -> (-5.575, 6)
  arc A8 (-3.575, 8) -> (-5.575, 6) centre (-3.575, 6) ccw
  arc A9 (5.575, 6) -> (3.575, 8) centre (3.575, 6) ccw
  arc A10 (3.575, 2) -> (5.575, 4) centre (3.575, 4) ccw
  arc A11 (-5.575, 4) -> (-3.575, 2) centre (-3.575, 4) ccw
  point P0 (-20.05, 10)
  point P1 (20.05, 10)
  dimension "d234" = 2
  dimension "d235" = 2
  dimension "d236" = 2
  dimension "d238" = 21.4065
  dimension "d241" = 2
  dimension "d242" = 2
  dimension "d243" = 2
  dimension "d244" = 2
  dimension "d245" = 37.4065
  dimension "d246" = 2
  dimension "d249" = 2
  dimension "d250" = 11.15
  dimension "d251" = 5.575
  constraint horizontal L4
  constraint vertical L5
  constraint horizontal L6
  constraint vertical L7
  constraint horizontal L8
  constraint vertical L9
  constraint horizontal L10
  constraint vertical L11
  constraint tangent L4 A0
  constraint tangent L7 A0
  constraint tangent L7 A1
  constraint tangent L6 A1
  constraint equal A0 A1
  constraint tangent L6 A2
  constraint tangent L5 A2
  constraint equal A0 A2
  constraint tangent L5 A3
  constraint tangent L4 A3
  constraint equal A0 A3
  constraint tangent L11 A4
  constraint tangent L8 A4
  constraint tangent L8 A5
  constraint tangent L9 A5
  constraint equal A4 A5
  constraint tangent L9 A6
  constraint tangent L10 A6
  constraint equal A4 A6
  constraint tangent L10 A7
  constraint tangent L11 A7
  constraint equal A4 A7
  constraint horizontal L12
  constraint vertical L13
  constraint horizontal L14
  constraint vertical L15
  constraint tangent L15 A8
  constraint tangent L12 A8
  constraint tangent L12 A9
  constraint tangent L13 A9
  constraint equal A8 A9
  constraint tangent L13 A10
  constraint tangent L14 A10
  constraint equal A8 A10
  constraint tangent L14 A11
  constraint tangent L15 A11
  constraint equal A8 A11
  constraint horizontal A2.centre A11.centre
  constraint horizontal A4.centre A9.centre
  measures "d234" distance of L5 P0
  measures "d235" distance of L1 L4
  measures "d236" distance of L3 L6
  measures "d238" distance of L5 L7
  measures "d241" radius of A0
  measures "d242" distance of L11 P1
  measures "d243" distance of L1 L8
  measures "d244" distance of L3 L10
  measures "d245" distance of L9 L11
  measures "d246" radius of A4
  measures "d249" radius of A8
  measures "d250" distance of L13 L15
  measures "d251" distance of origin L15
extrude "Extrude31" cut sketch "Sketch27" against normal blind 7 contours L4 L5 L6 L7 A0 A1 A2 A3 | L8 L9 L10 L11 A4 A5 A6 A7 | L12 L13 L14 L15 A8 A9 A10 A11
sketch "Sketch28" plane through (0, 42.6, 0) normal (0, 1, 0) x (-1, 0, 0)
  line L0 (51.5, 0) -> (51.5, 10)
  line L1 (51.5, 10) -> (-67.5, 10)
  line L2 (-67.5, 10) -> (-67.5, 0)
  line L3 (-67.5, 0) -> (51.5, 0)
  line L4 (-57.4565, 8) -> (-24.05, 8)
  line L5 (-22.05, 6) -> (-22.05, 4)
  line L6 (-24.05, 2) -> (-57.4565, 2)
  line L7 (-59.4565, 4) -> (-59.4565, 6)
  line L8 (-3.575, 8) -> (3.575, 8)
  line L9 (5.575, 6) -> (5.575, 4)
  line L10 (3.575, 2) -> (-3.575, 2)
  line L11 (-5.575, 4) -> (-5.575, 6)
  line L12 (24.05, 8) -> (41.4565, 8)
  line L13 (43.4565, 6) -> (43.4565, 4)
  line L14 (41.4565, 2) -> (24.05, 2)
  line L15 (22.05, 4) -> (22.05, 6)
  arc A0 (-57.4565, 8) -> (-59.4565, 6) centre (-57.4565, 6) ccw
  arc A1 (-22.05, 6) -> (-24.05, 8) centre (-24.05, 6) ccw
  arc A2 (-24.05, 2) -> (-22.05, 4) centre (-24.05, 4) ccw
  arc A3 (-59.4565, 4) -> (-57.4565, 2) centre (-57.4565, 4) ccw
  arc A4 (-3.575, 8) -> (-5.575, 6) centre (-3.575, 6) ccw
  arc A5 (5.575, 6) -> (3.575, 8) centre (3.575, 6) ccw
  arc A6 (3.575, 2) -> (5.575, 4) centre (3.575, 4) ccw
  arc A7 (-5.575, 4) -> (-3.575, 2) centre (-3.575, 4) ccw
  arc A8 (24.05, 8) -> (22.05, 6) centre (24.05, 6) ccw
  arc A9 (43.4565, 6) -> (41.4565, 8) centre (41.4565, 6) ccw
  arc A10 (41.4565, 2) -> (43.4565, 4) centre (41.4565, 4) ccw
  arc A11 (22.05, 4) -> (24.05, 2) centre (24.05, 4) ccw
  point P0 (-20.05, 10)
  point P1 (20.05, 10)
  dimension "d256" = 2
  dimension "d257" = 2
  dimension "d258" = 2
  dimension "d259" = 37.4065
  dimension "d260" = 2
  dimension "d261" = 2
  dimension "d262" = 2
  dimension "d263" = 21.4065
  dimension "d264" = 2
  dimension "d265" = 11.15
  dimension "d266" = 5.575
  constraint horizontal L4
  constraint vertical L5
  constraint horizontal L6
  constraint vertical L7
  constraint horizontal L8
  constraint vertical L9
  constraint horizontal L10
  constraint vertical L11
  constraint horizontal L12
  constraint vertical L13
  constraint horizontal L14
  constraint vertical L15
  constraint tangent L7 A0
  constraint tangent L4 A0
  constraint tangent L4 A1
  constraint tangent L5 A1
  constraint equal A0 A1
  constraint tangent L5 A2
  constraint tangent L6 A2
  constraint equal A0 A2
  constraint tangent L6 A3
  constraint tangent L7 A3
  constraint equal A0 A3
  constraint tangent L11 A4
  constraint tangent L8 A4
  constraint tangent L8 A5
  constraint tangent L9 A5
  constraint equal A4 A5
  constraint tangent L9 A6
  constraint tangent L10 A6
  constraint equal A4 A6
  constraint tangent L10 A7
  constraint tangent L11 A7
  constraint equal A4 A7
  constraint tangent L15 A8
  constraint tangent L12 A8
  constraint tangent L12 A9
  constraint tangent L13 A9
  constraint equal A8 A9
  constraint tangent L13 A10
  constraint tangent L14 A10
  constraint equal A8 A10
  constraint tangent L14 A11
  constraint tangent L15 A11
  constraint equal A8 A11
  constraint horizontal A1.centre A4.centre
  constraint horizontal A2.centre A7.centre
  constraint horizontal A5.centre A8.centre
  constraint horizontal A6.centre A11.centre
  measures "d256" distance of L5 P0
  measures "d257" distance of L1 L4
  measures "d258" distance of L3 L6
  measures "d259" distance of L5 L7
  measures "d260" radius of A0
  measures "d261" radius of A4
  measures "d262" radius of A8
  measures "d263" distance of L13 L15
  measures "d264" distance of L15 P1
  measures "d265" distance of L9 L11
  measures "d266" distance of origin L9
extrude "Extrude32" cut sketch "Sketch28" against normal blind 7 contours L4 L5 L6 L7 A0 A1 A2 A3 | L8 L9 L10 L11 A4 A5 A6 A7 | L12 L13 L14 L15 A8 A9 A10 A11
sketch "Sketch29" plane through (0, -28.5, 0) normal (0, -1, 0) x (1, 0, 0)
  line L0 (-61.5, 0) -> (-61.5, 6.5)
  line L1 (-61.5, 6.5) -> (-72.5, 6.5)
  line L2 (-72.5, 6.5) -> (-72.5, 0)
  line L3 (-72.5, 0) -> (-61.5, 0)
  line L4 (-69.5, 4.5) -> (-62.5, 4.5)
  line L5 (-61.5, 3.5) -> (-61.5, 3)
  line L6 (-62.5, 2) -> (-69.5, 2)
  line L7 (-70.5, 3) -> (-70.5, 3.5)
  arc A0 (-69.5, 4.5) -> (-70.5, 3.5) centre (-69.5, 3.5) ccw
  arc A1 (-61.5, 3.5) -> (-62.5, 4.5) centre (-62.5, 3.5) ccw
  arc A2 (-62.5, 2) -> (-61.5, 3) centre (-62.5, 3) ccw
  arc A3 (-70.5, 3) -> (-69.5, 2) centre (-69.5, 3) ccw
  point P0 (-61.5, 6.5)
  point P1 (-59.5, 6.5)
  dimension "d270" = 2
  dimension "d271" = 2
  dimension "d272" = 2
  dimension "d273" = 1
  dimension "d274" = 2
  constraint horizontal L4
  constraint vertical L5
  constraint horizontal L6
  constraint vertical L7
  constraint tangent L7 A0
  constraint tangent L4 A0
  constraint tangent L4 A1
  constraint tangent L5 A1
  constraint equal A0 A1
  constraint tangent L5 A2
  constraint tangent L6 A2
  constraint equal A0 A2
  constraint tangent L6 A3
  constraint tangent L7 A3
  constraint equal A0 A3
  measures "d270" distance of L2 L7
  measures "d271" distance of L1 L4
  measures "d272" distance of L3 L6
  measures "d273" radius of A0
  measures "d274" distance of L5 P1
extrude "Extrude33" cut sketch "Sketch29" against normal blind 60 contours L0 L4 L5 L6 L7 A0 A1 A2 A3
equation "d2 = ( 145 / 2 ) * 1 mm"
equation "d4 = ( 57.1 / 2 ) * 1 mm"
equation "d82 = ( 57 / 2 ) * 1 mm"
equation "d153 = ( 3.5 / 2 ) * 1 mm"
equation "d161 = ( 4.85 / 2 ) * 1 mm + 2 mm"
equation "d162 = ( 4.85 / 2 ) * 1 mm + 2 mm"
equation "d178 = ( 7.087 / 2 ) * 1 mm + 2 mm"
equation "d179 = ( 7.087 / 2 ) * 1 mm + 2 mm"
equation "d208 = ( 36.1 / 2 ) * 1 mm"
equation "d215 = ( 4.85 / 2 ) * 1 mm + 2 mm"
equation "d216 = ( 4.85 / 2 ) * 1 mm + 2 mm"
equation "d221 = ( 4.85 / 2 ) * 1 mm + 2 mm"
equation "d222 = ( 4.85 / 2 ) * 1 mm + 2 mm"
equation "d230 = ( 36.1 / 2 ) * 1 mm"
equation "d251 = ( 11.15 / 2 ) * 1 mm"
equation "d266 = ( 11.15 / 2 ) * 1 mm"

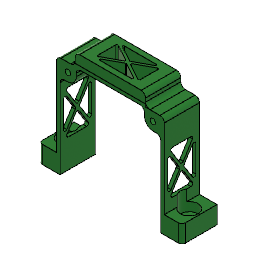
design "TM Front Holder"
Autodesk Fusion 360 part; units mm, degrees
sketch "Sketch1" plane through (0, 0, 0) normal (0, 0, 1) x (1, 0, 0)
  line L0 (28.55, 26.275) -> (30.55, 26.275)
  line L1 (30.55, 26.275) -> (30.55, -30.825)
  line L2 (30.55, -30.825) -> (28.55, -30.825)
  line L3 (28.55, -30.825) -> (28.55, 26.275)
  line L4 (-28.55, -30.825) -> (-30.55, -30.825)
  line L5 (-28.55, 26.275) -> (-28.55, -30.825)
  line L6 (-30.55, -30.825) -> (-30.55, 26.275)
  line L7 (-30.55, 26.275) -> (-28.55, 26.275)
  line L8 (-30.55, 26.275) -> (30.55, 26.275)
  line L9 (30.55, 26.275) -> (30.55, 28.275)
  line L10 (30.55, 28.275) -> (-30.55, 28.275)
  line L11 (-30.55, 28.275) -> (-30.55, 26.275)
  dimension "d1" = 2
  dimension "d4" = 26.275
  dimension "d5" = 2
  dimension "d7" = 57.1
  dimension "d8" = 28.55
  dimension "d9" = 2
  dimension "d99" = 59.1
  constraint horizontal L0
  constraint vertical L1
  constraint horizontal L2
  constraint vertical L3
  constraint horizontal L7
  constraint vertical L5
  constraint horizontal L4
  constraint vertical L6
  constraint horizontal L2.end L4.start
  constraint horizontal L8
  constraint vertical L9
  constraint horizontal L10
  constraint vertical L11
  constraint vertical L0.end L9.end
  measures "d1" distance of L1 L3
  measures "d4" distance of origin L0
  measures "d5" distance of L5 L6
  measures "d7" distance of L3 L5
  measures "d8" distance of origin L5
  measures "d9" distance of L8 L10
  measures "d99" distance of L2 L10
extrude "Extrude1" add sketch "Sketch1" along normal blind 20
sketch "Sketch2" plane through (0, 0, 20) normal (0, 0, 1) x (-1, 0, 0)
  line L0 (-30.55, 30.825) -> (-30.55, -28.275)
  line L1 (-30.55, -28.275) -> (30.55, -28.275)
  line L2 (30.55, -28.275) -> (30.55, 30.825)
  line L3 (30.55, 30.825) -> (28.55, 30.825)
  line L4 (28.55, 30.825) -> (28.55, -26.275)
  line L5 (28.55, -26.275) -> (-28.55, -26.275)
  line L6 (-28.55, -26.275) -> (-28.55, 30.825)
  line L7 (-28.55, 30.825) -> (-30.55, 30.825)
  line L8 (-30.55, 30.825) -> (-40.55, 30.825)
  line L9 (-40.55, 30.825) -> (-40.55, 28.325)
  line L10 (-40.55, 28.325) -> (-30.55, 28.325)
  line L11 (-30.55, 28.325) -> (-30.55, 30.825)
  line L12 (30.55, 30.825) -> (40.55, 30.825)
  line L13 (40.55, 30.825) -> (40.55, 28.325)
  line L14 (40.55, 28.325) -> (30.55, 28.325)
  line L15 (30.55, 28.325) -> (30.55, 30.825)
  dimension "d12" = 2.5
  dimension "d13" = 10
  dimension "d14" = 2.5
  dimension "d15" = 10
  constraint horizontal L8
  constraint vertical L9
  constraint horizontal L10
  constraint vertical L11
  constraint coincident L0.start L7.end
  constraint horizontal L12
  constraint vertical L13
  constraint horizontal L14
  constraint vertical L15
  constraint coincident L2.end L3.start
  measures "d12" distance of L8 L10
  measures "d13" distance of L9 L11
  measures "d14" distance of L12 L14
  measures "d15" distance of L13 L15
extrude "Extrude2" add sketch "Sketch2" against normal blind 20 contours L0 L8 L9 L10 L11 | L2 L12 L13 L14 L15
sketch "Sketch5" plane through (0, 28.275, 0) normal (0, 1, 0) x (-1, 0, 0)
  line L0 (-30.55, 0) -> (30.55, 0)
  line L1 (30.55, 0) -> (30.55, 20)
  line L2 (30.55, 20) -> (-30.55, 20)
  line L3 (-30.55, 20) -> (-30.55, 0)
  line L4 (-20, 20) -> (20, 20)
  line L5 (20, 20) -> (20, 0)
  line L6 (20, 0) -> (-20, 0)
  line L7 (-20, 0) -> (-20, 20)
  dimension "d32" = 40
  dimension "d96" = 20
  constraint horizontal L4
  constraint vertical L5
  constraint horizontal L6
  constraint vertical L7
  constraint coincident L0 L5.end
  constraint coincident L2 L4.start
  measures "d32" distance of L5 L7
  measures "d96" distance of origin L7
extrude "Extrude4" add sketch "Sketch5" along normal blind 10 contours L0 L2 L4 L5 L6 L7
sketch "Sketch6" plane through (0, 0, 0) normal (0, 0, -1) x (1, 0, 0)
  line L0 (20, -38.275) -> (20, -28.275)
  line L1 (-30.55, -28.275) -> (-20, -28.275)
  line L2 (30.55, -28.275) -> (30.55, 28.325)
  line L3 (30.55, 28.325) -> (40.55, 28.325)
  line L4 (40.55, 30.825) -> (28.55, 30.825)
  line L5 (28.55, 30.825) -> (28.55, -26.275)
  line L6 (28.55, -26.275) -> (-28.55, -26.275)
  line L7 (-28.55, -26.275) -> (-28.55, 30.825)
  line L8 (-28.55, 30.825) -> (-40.55, 30.825)
  line L9 (-40.55, 28.325) -> (-30.55, 28.325)
  line L10 (-30.55, 28.325) -> (-30.55, -28.275)
  line L11 (-20, -28.275) -> (-20, -38.275)
  line L12 (-20, -38.275) -> (20, -38.275)
  line L13 (-28.55, -26.275) -> (-19.3, -26.275)
  line L14 (-19.3, -23.775) -> (-19.3, -22.025)
  line L15 (-24.3, -17.025) -> (-26.05, -17.025)
  line L16 (-28.55, -17.025) -> (-28.55, -26.275)
  line L17 (28.55, -26.275) -> (19.3, -26.275)
  line L18 (19.3, -23.775) -> (19.3, -22.025)
  line L19 (24.3, -17.025) -> (26.05, -17.025)
  line L20 (28.55, -17.025) -> (28.55, -26.275)
  arc A0 (-19.3, -22.025) -> (-24.3, -17.025) centre (-24.3, -22.025) ccw
  arc A1 (24.3, -17.025) -> (19.3, -22.025) centre (24.3, -22.025) ccw
  line L21 (28.55, -14.525) -> (28.55, -10)
  line L22 (-28.55, -14.525) -> (-28.55, -10)
  arc A2 (26.05, -17.025) -> (28.55, -14.525) centre (26.05, -14.525) ccw
  arc A3 (-28.55, -14.525) -> (-26.05, -17.025) centre (-26.05, -14.525) ccw
  line L23 (16.8, -26.275) -> (13, -26.275)
  line L24 (-16.8, -26.275) -> (-13, -26.275)
  arc A4 (16.8, -26.275) -> (19.3, -23.775) centre (16.8, -23.775) ccw
  arc A5 (-19.3, -23.775) -> (-16.8, -26.275) centre (-16.8, -23.775) ccw
  line L25 (20, -28.275) -> (30.55, -28.275)
  line L26 (-40.55, 30.825) -> (-40.55, 28.325)
  line L27 (40.55, 28.325) -> (40.55, 30.825)
  dimension "d38" = 9.25
  dimension "d39" = 9.25
  dimension "d40" = 9.25
  dimension "d41" = 9.25
  dimension "d42" = 5
  dimension "d43" = 5
  dimension "d44" = 2.5
  dimension "d45" = 2.5
  dimension "d46" = 2.5
  dimension "d47" = 2.5
  constraint horizontal L13
  constraint vertical L14
  constraint horizontal L15
  constraint vertical L16
  constraint coincident L6.end L7.start
  constraint horizontal L17
  constraint vertical L18
  constraint horizontal L19
  constraint vertical L20
  constraint coincident L5.end L6.start
  constraint tangent L15 A0
  constraint tangent L14 A0
  constraint tangent L19 A1
  constraint tangent L18 A1
  constraint coincident L5 L21.end
  constraint coincident L7 L22.end
  constraint coincident L20.start L19
  constraint coincident L20.start L21
  constraint tangent L19 A2
  constraint tangent L21 A2
  constraint coincident L16.start L22
  constraint coincident L16.start L15
  constraint tangent L22 A3
  constraint tangent L15 A3
  constraint coincident L6 L23.end
  constraint coincident L6 L24.end
  constraint coincident L17.end L23
  constraint coincident L17.end L18
  constraint tangent L23 A4
  constraint tangent L18 A4
  constraint coincident L13.end L24
  constraint coincident L13.end L14
  constraint tangent L24 A5
  constraint tangent L14 A5
  measures "d38" distance of L14 L16
  measures "d39" distance of L13 L15
  measures "d40" distance of L18 L20
  measures "d41" distance of L17 L19
  measures "d42" radius of A0
  measures "d43" radius of A1
  measures "d44" radius of A2
  measures "d45" radius of A3
  measures "d46" radius of A4
  measures "d47" radius of A5
extrude "Extrude5" add sketch "Sketch6" against normal blind 20 contours L5 L6 L17 L18 L19 L20 A1 A2 A4 | L6 L7 L13 L14 L15 L16 A0 A3 A5
sketch "Sketch7" plane through (0, 0, 20) normal (0, 0, 1) x (-1, 0, 0)
  line L0 (-30.55, -28.275) -> (-20, -28.275)
  line L1 (-20, -28.275) -> (20, -28.275)
  line L2 (30.55, -28.275) -> (30.55, 28.325)
  line L3 (30.55, 28.325) -> (40.55, 28.325)
  line L4 (40.55, 28.325) -> (40.55, 30.825)
  line L5 (40.55, 30.825) -> (28.55, 30.825)
  line L6 (28.55, 30.825) -> (28.55, -14.525)
  arc A0 (26.05, -17.025) -> (28.55, -14.525) centre (26.05, -14.525) ccw
  line L7 (26.05, -17.025) -> (24.3, -17.025)
  arc A1 (24.3, -17.025) -> (19.3, -22.025) centre (24.3, -22.025) ccw
  line L8 (19.3, -22.025) -> (19.3, -23.775)
  arc A2 (16.8, -26.275) -> (19.3, -23.775) centre (16.8, -23.775) ccw
  line L9 (16.8, -26.275) -> (-16.8, -26.275)
  arc A3 (-19.3, -23.775) -> (-16.8, -26.275) centre (-16.8, -23.775) ccw
  line L10 (-19.3, -23.775) -> (-19.3, -22.025)
  arc A4 (-19.3, -22.025) -> (-24.3, -17.025) centre (-24.3, -22.025) ccw
  line L11 (-24.3, -17.025) -> (-26.05, -17.025)
  arc A5 (-28.55, -14.525) -> (-26.05, -17.025) centre (-26.05, -14.525) ccw
  line L12 (-28.55, -14.525) -> (-28.55, 30.825)
  line L13 (-28.55, 30.825) -> (-40.55, 30.825)
  line L14 (-40.55, 30.825) -> (-40.55, 28.325)
  line L15 (-40.55, 28.325) -> (-30.55, 28.325)
  line L16 (-30.55, 28.325) -> (-30.55, -28.275)
  line L17 (20, -28.275) -> (30.55, -28.275)
  point P0 (24.05, -21.775)
  point P1 (-24.05, -21.775)
  dimension "d52" = 6.5
  dimension "d54" = 6.5
  constraint horizontal P0 P1
  measures "d52" distance of L2 P0
  measures "d54" distance of L16 P1
hole "Hole2" at (-24.05, 21.775, 20) at (24.05, 21.775, 20) direction (0, 0, -1) diameter 3 end through all
sketch "Sketch9" plane through (0, 38.275, 0) normal (0, 1, 0) x (-1, 0, 0)
  line L0 (-20, 0) -> (20, 0)
  line L1 (20, 20) -> (-20, 20)
  line L2 (-9.0392, 17) -> (9.0392, 17)
  line L3 (-9.0392, 3) -> (9.0392, 3)
  line L4 (-12, 15.1577) -> (-12, 4.8423)
  line L5 (12, 15.1577) -> (12, 4.8399)
  line L6 (-9.2786, 3.9389) -> (-0.2394, 8.8694)
  line L7 (-11.2606, 4.4033) -> (-1.8047, 9.5611)
  line L8 (-1.8047, 10.4389) -> (-11.2606, 15.5967)
  line L9 (11.2606, 15.5967) -> (1.7742, 10.4223)
  line L10 (-9.2786, 16.0611) -> (-0.2394, 11.1306)
  line L11 (0.2394, 11.1306) -> (9.2786, 16.0611)
  line L12 (0.2394, 8.8694) -> (9.2786, 3.9389)
  line L13 (1.7753, 9.5438) -> (11.2617, 4.4003)
  arc A0 (-11.2606, 15.5967) -> (-12, 15.1577) centre (-11.5, 15.1577) ccw
  arc A1 (-1.8047, 9.5611) -> (-1.8047, 10.4389) centre (-2.0442, 10) ccw
  arc A2 (-12, 4.8423) -> (-11.2606, 4.4033) centre (-11.5, 4.8423) ccw
  arc A3 (-9.2786, 3.9389) -> (-9.0392, 3) centre (-9.0392, 3.5) ccw
  arc A4 (0.2394, 8.8694) -> (-0.2394, 8.8694) centre (0, 8.4305) ccw
  arc A5 (9.0392, 3) -> (9.2786, 3.9389) centre (9.0392, 3.5) ccw
  arc A6 (11.2617, 4.4003) -> (12, 4.8399) centre (11.5, 4.8399) ccw
  arc A7 (1.7742, 10.4223) -> (1.7753, 9.5438) centre (2.0137, 9.9834) ccw
  arc A8 (12, 15.1577) -> (11.2606, 15.5967) centre (11.5, 15.1577) ccw
  arc A9 (9.2786, 16.0611) -> (9.0392, 17) centre (9.0392, 16.5) ccw
  arc A10 (-9.0392, 17) -> (-9.2786, 16.0611) centre (-9.0392, 16.5) ccw
  arc A11 (-0.2394, 11.1306) -> (0.2394, 11.1306) centre (0, 11.5695) ccw
  line L14 (20, 0) -> (20, 20)
  line L15 (-20, 20) -> (-20, 0)
  point P0 (11, 17)
  point P1 (12, 16)
  point P2 (0, 10)
  dimension "d60" = 11
  dimension "d61" = 6
  dimension "d62" = 0.5
  constraint horizontal L3
  constraint vertical L4
  constraint vertical L5
  constraint parallel L7 L9
  constraint tangent L4 A0
  constraint tangent L8 A0
  constraint tangent L8 A1
  constraint tangent L7 A1
  constraint equal A0 A1
  constraint tangent L4 A2
  constraint tangent L7 A2
  constraint equal A0 A2
  constraint tangent L3 A3
  constraint tangent L6 A3
  constraint equal A0 A3
  constraint tangent L12 A4
  constraint tangent L6 A4
  constraint equal A0 A4
  constraint tangent L12 A5
  constraint tangent L3 A5
  constraint equal A0 A5
  constraint tangent L13 A6
  constraint tangent L5 A6
  constraint equal A0 A6
  constraint tangent L9 A7
  constraint tangent L13 A7
  constraint equal A0 A7
  constraint coincident P1 L5
  constraint coincident P1 L9
  constraint tangent L5 A8
  constraint tangent L9 A8
  constraint equal A0 A8
  constraint coincident P0 L11
  constraint tangent L11 A9
  constraint tangent L2 A9
  constraint equal A0 A9
  constraint tangent L2 A10
  constraint tangent L10 A10
  constraint equal A0 A10
  constraint tangent L11 A11
  constraint tangent L10 A11
  constraint equal A0 A11
  measures "d60" horizontal distance of P0 P2
  measures "d61" vertical distance of P1 P2
  measures "d62" radius of A0
extrude "Extrude7" cut sketch "Sketch9" against normal blind 15 contours L2 L10 L11 A9 A10 A11 | L3 L6 L12 A3 A4 A5 | L4 L7 L8 A0 A1 A2 | L5 L9 L13 A6 A7 A8